Autodesk Fusion 360 part; units mm, degrees
(part 2 of 4)
sketch "sketch 3732" plane through (0, 0, 0) normal (0, 1, 0) x (1, 0, 0)
  arc A0 (-1.8258, -74.9829) -> (1.8258, -74.9829) centre (0, 0) ccw
  arc A1 (9.805, -63.395) -> (9.351, -63.0605) centre (9.4097, -63.4561) ccw
  line L0 (4.6702, -65.7139) -> (4.5475, -63.9874)
  arc A2 (14.9052, -73.5092) -> (18.4653, -72.6966) centre (0, 0) ccw
  spline S0 degree 3 poles (4.376, -68.1369) (4.6576, -66.7896) (4.6745, -65.9819) (4.6702, -65.7139) knots 0 0 0 0 1 1 1 1
  line L1 (9.805, -63.395) -> (10.0696, -65.1055)
  spline S1 degree 3 poles (10.8935, -67.4001) (11.5834, -68.8958) (12.799, -71.009) (14.9052, -73.5092) knots 0 0 0 0 1 1 1 1
  spline S2 degree 3 poles (10.0696, -65.1055) (10.1251, -65.3677) (10.3212, -66.1515) (10.8935, -67.4001) knots 0 0 0 0 1 1 1 1
  arc A3 (4.9157, -63.5602) -> (9.351, -63.0605) centre (0, 0) ccw
  spline S3 degree 3 poles (-4.3775, -68.1342) (-4.0378, -69.746) (-3.3229, -72.0767) (-1.8258, -74.9829) knots 0 0 0 0 1 1 1 1
  spline S4 degree 3 poles (1.8258, -74.9829) (3.3229, -72.0767) (4.0378, -69.746) (4.376, -68.1369) knots 0 0 0 0 1 1 1 1
  arc A4 (4.9157, -63.5602) -> (4.5475, -63.9874) centre (4.9465, -63.959) ccw
  arc A5 (45.3236, -59.7623) -> (48.1785, -57.4856) centre (0, 0) ccw
  spline S5 degree 3 poles (19.4282, -65.4548) (19.403, -64.0786) (19.2396, -63.2874) (19.1758, -63.0271) knots 0 0 0 0 1 1 1 1
  arc A6 (43.4724, -46.6285) -> (46.6285, -43.4724) centre (0, 0) ccw
  spline S6 degree 3 poles (48.4653, -44.6233) (48.6722, -44.7937) (49.3142, -45.2841) (50.5402, -45.9035) knots 0 0 0 0 1 1 1 1
  arc A7 (18.9359, -60.8728) -> (18.672, -61.3711) centre (19.0547, -61.2547) ccw
  line L2 (32.7199, -57.1798) -> (31.8603, -55.6775)
  line L3 (47.192, -43.4509) -> (48.4653, -44.6233)
  spline S7 degree 3 poles (50.5402, -45.9035) (52.0121, -46.6428) (54.28, -47.537) (57.4856, -48.1785) knots 0 0 0 0 1 1 1 1
  arc A8 (57.4856, -48.1785) -> (59.7623, -45.3236) centre (0, 0) ccw
  line L4 (55.6775, -31.8603) -> (57.1798, -32.7199)
  spline S8 degree 3 poles (24.3045, -61.2325) (24.4169, -61.4758) (24.7825, -62.1962) (25.6183, -63.2862) knots 0 0 0 0 1 1 1 1
  arc A9 (30.8888, -68.3494) -> (34.1789, -66.765) centre (0, 0) ccw
  arc A10 (18.9359, -60.8728) -> (23.1489, -59.3986) centre (0, 0) ccw
  line L5 (23.6659, -59.6237) -> (24.3045, -61.2325)
  spline S9 degree 3 poles (25.6183, -63.2862) (26.6237, -64.5909) (28.2791, -66.3806) (30.8888, -68.3494) knots 0 0 0 0 1 1 1 1
  spline S10 degree 3 poles (18.4653, -72.6966) (19.2781, -69.5301) (19.4565, -67.0988) (19.4282, -65.4548) knots 0 0 0 0 1 1 1 1
  spline S11 degree 3 poles (34.1789, -66.765) (34.2667, -63.4971) (33.8996, -61.087) (33.5061, -59.4906) knots 0 0 0 0 1 1 1 1
  arc A11 (36.3401, -52.8627) -> (35.7859, -52.7582) centre (36.0104, -53.0893) ccw
  spline S12 degree 3 poles (39.0585, -55.9988) (40.329, -57.0472) (42.3411, -58.4236) (45.3236, -59.7623) knots 0 0 0 0 1 1 1 1
  arc A12 (47.192, -43.4509) -> (46.6285, -43.4724) centre (46.9211, -43.7451) ccw
  spline S13 degree 3 poles (37.3206, -54.289) (37.4844, -54.5012) (38.0011, -55.1222) (39.0585, -55.9988) knots 0 0 0 0 1 1 1 1
  arc A13 (32.0066, -55.1329) -> (35.7859, -52.7582) centre (0, 0) ccw
  line L6 (44.6233, -48.4653) -> (43.4509, -47.192)
  arc A14 (43.4724, -46.6285) -> (43.4509, -47.192) centre (43.7451, -46.9211) ccw
  spline S14 degree 3 poles (48.1785, -57.4856) (47.537, -54.28) (46.6428, -52.0121) (45.904, -50.5432) knots 0 0 0 0 1 1 1 1
  line L7 (19.1758, -63.0271) -> (18.672, -61.3711)
  arc A15 (23.6659, -59.6237) -> (23.1489, -59.3986) centre (23.2941, -59.7713) ccw
  arc A16 (32.0066, -55.1329) -> (31.8603, -55.6775) centre (32.2074, -55.4789) ccw
  spline S15 degree 3 poles (33.5061, -59.4906) (33.1753, -58.1545) (32.84, -57.4195) (32.7199, -57.1798) knots 0 0 0 0 1 1 1 1
  line L8 (36.3401, -52.8627) -> (37.3206, -54.289)
  spline S16 degree 3 poles (45.904, -50.5432) (45.2841, -49.3142) (44.7937, -48.6722) (44.6233, -48.4653) knots 0 0 0 0 1 1 1 1
  line L9 (54.289, -37.3206) -> (52.8627, -36.3401)
  spline S17 degree 3 poles (59.4875, -33.5063) (61.087, -33.8996) (63.4971, -34.2667) (66.765, -34.1789) knots 0 0 0 0 1 1 1 1
  spline S18 degree 3 poles (68.3494, -30.8888) (66.3806, -28.2791) (64.5909, -26.6237) (63.2879, -25.6209) knots 0 0 0 0 1 1 1 1
  arc A17 (59.3986, -23.1489) -> (60.8728, -18.9359) centre (0, 0) ccw
  line L10 (61.2325, -24.3045) -> (59.6237, -23.6659)
  line L11 (61.3711, -18.672) -> (63.0271, -19.1758)
  spline S19 degree 3 poles (56, -39.0614) (55.1222, -38.0011) (54.5012, -37.4844) (54.289, -37.3206) knots 0 0 0 0 1 1 1 1
  spline S20 degree 3 poles (63.0271, -19.1758) (63.2874, -19.2396) (64.0786, -19.403) (65.4519, -19.4291) knots 0 0 0 0 1 1 1 1
  spline S21 degree 3 poles (65.4519, -19.4291) (67.0988, -19.4565) (69.5301, -19.2781) (72.6966, -18.4653) knots 0 0 0 0 1 1 1 1
  arc A18 (72.6966, -18.4653) -> (73.5092, -14.9052) centre (0, 0) ccw
  arc A19 (63.0605, -9.351) -> (63.5602, -4.9157) centre (0, 0) ccw
  arc A20 (52.7582, -35.7859) -> (55.1329, -32.0066) centre (0, 0) ccw
  arc A21 (63.0605, -9.351) -> (63.395, -9.805) centre (63.4561, -9.4097) ccw
  arc A22 (52.7582, -35.7859) -> (52.8627, -36.3401) centre (53.0893, -36.0104) ccw
  line L12 (65.1055, -10.0696) -> (63.395, -9.805)
  spline S22 degree 3 poles (59.7623, -45.3236) (58.4236, -42.3411) (57.0472, -40.329) (56, -39.0614) knots 0 0 0 0 1 1 1 1
  arc A23 (55.6775, -31.8603) -> (55.1329, -32.0066) centre (55.4789, -32.2074) ccw
  spline S23 degree 3 poles (57.1798, -32.7199) (57.4195, -32.84) (58.1545, -33.1753) (59.4875, -33.5063) knots 0 0 0 0 1 1 1 1
  spline S24 degree 3 poles (63.2879, -25.6209) (62.1962, -24.7825) (61.4758, -24.4169) (61.2325, -24.3045) knots 0 0 0 0 1 1 1 1
  arc A24 (66.765, -34.1789) -> (68.3494, -30.8888) centre (0, 0) ccw
  arc A25 (59.3986, -23.1489) -> (59.6237, -23.6659) centre (59.7713, -23.2941) ccw
  arc A26 (61.3711, -18.672) -> (60.8728, -18.9359) centre (61.2547, -19.0547) ccw
  spline S25 degree 3 poles (-10.0696, 65.1055) (-10.1251, 65.3677) (-10.3212, 66.1515) (-10.8935, 67.4001) knots 0 0 0 0 1 1 1 1
  spline S26 degree 3 poles (19.1758, 63.0271) (19.2396, 63.2874) (19.403, 64.0786) (19.4291, 65.4519) knots 0 0 0 0 1 1 1 1
  arc A27 (9.351, 63.0605) -> (4.9157, 63.5602) centre (0, 0) ccw
  arc A28 (-36.3401, 52.8627) -> (-35.7859, 52.7582) centre (-36.0104, 53.0893) ccw
  line L13 (-32.7199, 57.1798) -> (-31.8603, 55.6775)
  arc A29 (-9.805, 63.395) -> (-9.351, 63.0605) centre (-9.4097, 63.4561) ccw
  arc A30 (-32.0066, 55.1329) -> (-31.8603, 55.6775) centre (-32.2074, 55.4789) ccw
  arc A31 (34.1789, 66.765) -> (30.8888, 68.3494) centre (0, 0) ccw
  spline S27 degree 3 poles (-10.8935, 67.4001) (-11.5834, 68.8958) (-12.799, 71.009) (-14.9052, 73.5092) knots 0 0 0 0 1 1 1 1
  arc A32 (18.672, 61.3711) -> (18.9359, 60.8728) centre (19.0547, 61.2547) ccw
  line L14 (-4.6702, 65.7139) -> (-4.5475, 63.9874)
  arc A33 (-18.9359, 60.8728) -> (-23.1489, 59.3986) centre (0, 0) ccw
  spline S28 degree 3 poles (19.4291, 65.4519) (19.4565, 67.0988) (19.2781, 69.5301) (18.4653, 72.6966) knots 0 0 0 0 1 1 1 1
  spline S29 degree 3 poles (-34.1789, 66.765) (-34.2667, 63.4971) (-33.8996, 61.087) (-33.5061, 59.4906) knots 0 0 0 0 1 1 1 1
  arc A34 (-45.3236, 59.7623) -> (-48.1785, 57.4856) centre (0, 0) ccw
  spline S30 degree 3 poles (-45.904, 50.5432) (-45.2841, 49.3142) (-44.7937, 48.6722) (-44.6233, 48.4653) knots 0 0 0 0 1 1 1 1
  arc A35 (-14.9052, 73.5092) -> (-18.4653, 72.6966) centre (0, 0) ccw
  spline S31 degree 3 poles (10.8956, 67.4023) (10.3212, 66.1515) (10.1251, 65.3677) (10.0696, 65.1055) knots 0 0 0 0 1 1 1 1
  spline S32 degree 3 poles (14.9052, 73.5092) (12.799, 71.009) (11.5834, 68.8958) (10.8956, 67.4023) knots 0 0 0 0 1 1 1 1
  spline S33 degree 3 poles (-37.3206, 54.289) (-37.4844, 54.5012) (-38.0011, 55.1222) (-39.0585, 55.9988) knots 0 0 0 0 1 1 1 1
  spline S34 degree 3 poles (-1.8258, 74.9829) (-3.3229, 72.0767) (-4.0378, 69.746) (-4.376, 68.1369) knots 0 0 0 0 1 1 1 1
  line L15 (-47.192, 43.4509) -> (-48.4653, 44.6233)
  arc A36 (-43.4724, 46.6285) -> (-46.6285, 43.4724) centre (0, 0) ccw
  arc A37 (-47.192, 43.4509) -> (-46.6285, 43.4724) centre (-46.9211, 43.7451) ccw
  spline S35 degree 3 poles (-18.4653, 72.6966) (-19.2781, 69.5301) (-19.4565, 67.0988) (-19.4282, 65.4548) knots 0 0 0 0 1 1 1 1
  spline S36 degree 3 poles (4.3775, 68.1342) (4.0378, 69.746) (3.3229, 72.0767) (1.8258, 74.9829) knots 0 0 0 0 1 1 1 1
  arc A38 (23.1489, 59.3986) -> (23.6659, 59.6237) centre (23.2941, 59.7713) ccw
  line L16 (4.5475, 63.9874) -> (4.6702, 65.7139)
  spline S37 degree 3 poles (-33.5061, 59.4906) (-33.1753, 58.1545) (-32.84, 57.4195) (-32.7199, 57.1798) knots 0 0 0 0 1 1 1 1
  arc A39 (4.5475, 63.9874) -> (4.9157, 63.5602) centre (4.9465, 63.959) ccw
  spline S38 degree 3 poles (-24.3045, 61.2325) (-24.4169, 61.4758) (-24.7825, 62.1962) (-25.6183, 63.2862) knots 0 0 0 0 1 1 1 1
  circle A40 centre (0, 0) radius 4
  arc A41 (-4.9157, 63.5602) -> (-4.5475, 63.9874) centre (-4.9465, 63.959) ccw
  arc A42 (-32.0066, 55.1329) -> (-35.7859, 52.7582) centre (0, 0) ccw
  line L17 (-36.3401, 52.8627) -> (-37.3206, 54.289)
  spline S39 degree 3 poles (-39.0585, 55.9988) (-40.329, 57.0472) (-42.3411, 58.4236) (-45.3236, 59.7623) knots 0 0 0 0 1 1 1 1
  spline S40 degree 3 poles (33.5063, 59.4875) (33.8996, 61.087) (34.2667, 63.4971) (34.1789, 66.765) knots 0 0 0 0 1 1 1 1
  arc A43 (-23.6659, 59.6237) -> (-23.1489, 59.3986) centre (-23.2941, 59.7713) ccw
  arc A44 (-30.8888, 68.3494) -> (-34.1789, 66.765) centre (0, 0) ccw
  arc A45 (-18.9359, 60.8728) -> (-18.672, 61.3711) centre (-19.0547, 61.2547) ccw
  arc A46 (23.1489, 59.3986) -> (18.9359, 60.8728) centre (0, 0) ccw
  arc A47 (-4.9157, 63.5602) -> (-9.351, 63.0605) centre (0, 0) ccw
  spline S41 degree 3 poles (-25.6183, 63.2862) (-26.6237, 64.5909) (-28.2791, 66.3806) (-30.8888, 68.3494) knots 0 0 0 0 1 1 1 1
  line L18 (-19.1758, 63.0271) -> (-18.672, 61.3711)
  line L19 (18.672, 61.3711) -> (19.1758, 63.0271)
  arc A48 (-43.4724, 46.6285) -> (-43.4509, 47.192) centre (-43.7451, 46.9211) ccw
  line L20 (-44.6233, 48.4653) -> (-43.4509, 47.192)
  line L21 (24.3045, 61.2325) -> (23.6659, 59.6237)
  spline S42 degree 3 poles (4.6702, 65.7139) (4.6745, 65.9819) (4.6576, 66.7896) (4.3775, 68.1342) knots 0 0 0 0 1 1 1 1
  spline S43 degree 3 poles (-4.376, 68.1369) (-4.6576, 66.7896) (-4.6745, 65.9819) (-4.6702, 65.7139) knots 0 0 0 0 1 1 1 1
  spline S44 degree 3 poles (-19.4282, 65.4548) (-19.403, 64.0786) (-19.2396, 63.2874) (-19.1758, 63.0271) knots 0 0 0 0 1 1 1 1
  spline S45 degree 3 poles (-48.1785, 57.4856) (-47.537, 54.28) (-46.6428, 52.0121) (-45.904, 50.5432) knots 0 0 0 0 1 1 1 1
  spline S46 degree 3 poles (67.4023, -10.8956) (66.1515, -10.3212) (65.3677, -10.1251) (65.1055, -10.0696) knots 0 0 0 0 1 1 1 1
  arc A49 (18.4653, 72.6966) -> (14.9052, 73.5092) centre (0, 0) ccw
  line L22 (-9.805, 63.395) -> (-10.0696, 65.1055)
  line L23 (10.0696, 65.1055) -> (9.805, 63.395)
  spline S47 degree 3 poles (-4.6702, -65.7139) (-4.6745, -65.9819) (-4.6576, -66.7896) (-4.3775, -68.1342) knots 0 0 0 0 1 1 1 1
  arc A50 (9.351, 63.0605) -> (9.805, 63.395) centre (9.4097, 63.4561) ccw
  spline S48 degree 3 poles (30.8888, 68.3494) (28.2791, 66.3806) (26.6237, 64.5909) (25.6209, 63.2879) knots 0 0 0 0 1 1 1 1
  spline S49 degree 3 poles (32.7199, 57.1798) (32.84, 57.4195) (33.1753, 58.1545) (33.5063, 59.4875) knots 0 0 0 0 1 1 1 1
  line L24 (-23.6659, 59.6237) -> (-24.3045, 61.2325)
  spline S50 degree 3 poles (25.6209, 63.2879) (24.7825, 62.1962) (24.4169, 61.4758) (24.3045, 61.2325) knots 0 0 0 0 1 1 1 1
  spline S51 degree 3 poles (73.5092, -14.9052) (71.009, -12.799) (68.8958, -11.5834) (67.4023, -10.8956) knots 0 0 0 0 1 1 1 1
  arc A51 (1.8258, 74.9829) -> (-1.8258, 74.9829) centre (0, 0) ccw
  spline S52 degree 3 poles (-68.1369, -4.376) (-66.7896, -4.6576) (-65.9819, -4.6745) (-65.7139, -4.6702) knots 0 0 0 0 1 1 1 1
  line L25 (-63.395, -9.805) -> (-65.1055, -10.0696)
  arc A52 (-63.0605, 9.351) -> (-63.5602, 4.9157) centre (0, 0) ccw
  arc A53 (-59.6237, -23.6659) -> (-59.3986, -23.1489) centre (-59.7713, -23.2941) ccw
  arc A54 (-55.1329, -32.0066) -> (-52.7582, -35.7859) centre (0, 0) ccw
  arc A55 (-52.8627, -36.3401) -> (-52.7582, -35.7859) centre (-53.0893, -36.0104) ccw
  line L26 (-52.8627, -36.3401) -> (-54.289, -37.3206)
  spline S53 degree 3 poles (-65.4519, 19.4291) (-67.0988, 19.4565) (-69.5301, 19.2781) (-72.6966, 18.4653) knots 0 0 0 0 1 1 1 1
  spline S54 degree 3 poles (-73.5092, 14.9052) (-71.009, 12.799) (-68.8958, 11.5834) (-67.4023, 10.8956) knots 0 0 0 0 1 1 1 1
  arc A56 (-52.7582, 35.7859) -> (-55.1329, 32.0066) centre (0, 0) ccw
  line L27 (-65.7139, -4.6702) -> (-63.9874, -4.5475)
  arc A57 (-57.4856, 48.1785) -> (-59.7623, 45.3236) centre (0, 0) ccw
  arc A58 (-59.3986, 23.1489) -> (-59.6237, 23.6659) centre (-59.7713, 23.2941) ccw
  spline S55 degree 3 poles (-63.2879, 25.6209) (-62.1962, 24.7825) (-61.4758, 24.4169) (-61.2325, 24.3045) knots 0 0 0 0 1 1 1 1
  line L28 (-61.3711, 18.672) -> (-63.0271, 19.1758)
  spline S56 degree 3 poles (-54.289, -37.3206) (-54.5012, -37.4844) (-55.1222, -38.0011) (-55.9988, -39.0585) knots 0 0 0 0 1 1 1 1
  arc A59 (-59.7623, -45.3236) -> (-57.4856, -48.1785) centre (0, 0) ccw
  spline S57 degree 3 poles (-55.9988, -39.0585) (-57.0472, -40.329) (-58.4236, -42.3411) (-59.7623, -45.3236) knots 0 0 0 0 1 1 1 1
  arc A60 (-63.0605, 9.351) -> (-63.395, 9.805) centre (-63.4561, 9.4097) ccw
  spline S58 degree 3 poles (-65.1055, -10.0696) (-65.3677, -10.1251) (-66.1515, -10.3212) (-67.4001, -10.8935) knots 0 0 0 0 1 1 1 1
  arc A61 (-61.3711, 18.672) -> (-60.8728, 18.9359) centre (-61.2547, 19.0547) ccw
  spline S59 degree 3 poles (-63.0271, 19.1758) (-63.2874, 19.2396) (-64.0786, 19.403) (-65.4519, 19.4291) knots 0 0 0 0 1 1 1 1
  spline S60 degree 3 poles (-59.4875, 33.5063) (-61.087, 33.8996) (-63.4971, 34.2667) (-66.765, 34.1789) knots 0 0 0 0 1 1 1 1
  spline S61 degree 3 poles (-50.5402, 45.9035) (-52.0121, 46.6428) (-54.28, 47.537) (-57.4856, 48.1785) knots 0 0 0 0 1 1 1 1
  line L29 (-61.2325, 24.3045) -> (-59.6237, 23.6659)
  arc A62 (-55.6775, 31.8603) -> (-55.1329, 32.0066) centre (-55.4789, 32.2074) ccw
  spline S62 degree 3 poles (-65.7139, 4.6702) (-65.9819, 4.6745) (-66.7896, 4.6576) (-68.1342, 4.3775) knots 0 0 0 0 1 1 1 1
  arc A63 (-63.395, -9.805) -> (-63.0605, -9.351) centre (-63.4561, -9.4097) ccw
  line L30 (-65.1055, 10.0696) -> (-63.395, 9.805)
  spline S63 degree 3 poles (-67.4023, 10.8956) (-66.1515, 10.3212) (-65.3677, 10.1251) (-65.1055, 10.0696) knots 0 0 0 0 1 1 1 1
  arc A64 (-63.9874, 4.5475) -> (-63.5602, 4.9157) centre (-63.959, 4.9465) ccw
  arc A65 (-63.5602, -4.9157) -> (-63.0605, -9.351) centre (0, 0) ccw
  spline S64 degree 3 poles (-68.1342, 4.3775) (-69.746, 4.0378) (-72.0767, 3.3229) (-74.9829, 1.8258) knots 0 0 0 0 1 1 1 1
  line L31 (-63.9874, 4.5475) -> (-65.7139, 4.6702)
  line L32 (-57.1798, -32.7199) -> (-55.6775, -31.8603)
  spline S65 degree 3 poles (-66.765, -34.1789) (-63.4971, -34.2667) (-61.087, -33.8996) (-59.4906, -33.5061) knots 0 0 0 0 1 1 1 1
  arc A66 (-63.5602, -4.9157) -> (-63.9874, -4.5475) centre (-63.959, -4.9465) ccw
  arc A67 (-66.765, 34.1789) -> (-68.3494, 30.8888) centre (0, 0) ccw
  arc A68 (-60.8728, -18.9359) -> (-61.3711, -18.672) centre (-61.2547, -19.0547) ccw
  spline S66 degree 3 poles (-48.4653, 44.6233) (-48.6722, 44.7937) (-49.3142, 45.2841) (-50.5402, 45.9035) knots 0 0 0 0 1 1 1 1
  arc A69 (-60.8728, -18.9359) -> (-59.3986, -23.1489) centre (0, 0) ccw
  line L33 (-54.289, 37.3206) -> (-52.8627, 36.3401)
  spline S67 degree 3 poles (-72.6966, -18.4653) (-69.5301, -19.2781) (-67.0988, -19.4565) (-65.4548, -19.4282) knots 0 0 0 0 1 1 1 1
  arc A70 (-52.7582, 35.7859) -> (-52.8627, 36.3401) centre (-53.0893, 36.0104) ccw
  arc A71 (-73.5092, -14.9052) -> (-72.6966, -18.4653) centre (0, 0) ccw
  spline S68 degree 3 poles (-57.1798, 32.7199) (-57.4195, 32.84) (-58.1545, 33.1753) (-59.4875, 33.5063) knots 0 0 0 0 1 1 1 1
  line L34 (-59.6237, -23.6659) -> (-61.2325, -24.3045)
  arc A72 (-72.6966, 18.4653) -> (-73.5092, 14.9052) centre (0, 0) ccw
  spline S69 degree 3 poles (-74.9829, -1.8258) (-72.0767, -3.3229) (-69.746, -4.0378) (-68.1369, -4.376) knots 0 0 0 0 1 1 1 1
  line L35 (-55.6775, 31.8603) -> (-57.1798, 32.7199)
  spline S70 degree 3 poles (-67.4001, -10.8935) (-68.8958, -11.5834) (-71.009, -12.799) (-73.5092, -14.9052) knots 0 0 0 0 1 1 1 1
  spline S71 degree 3 poles (-56, 39.0614) (-55.1222, 38.0011) (-54.5012, 37.4844) (-54.289, 37.3206) knots 0 0 0 0 1 1 1 1
  spline S72 degree 3 poles (-65.4548, -19.4282) (-64.0786, -19.403) (-63.2874, -19.2396) (-63.0271, -19.1758) knots 0 0 0 0 1 1 1 1
  arc A73 (-74.9829, 1.8258) -> (-74.9829, -1.8258) centre (0, 0) ccw
  line L36 (-63.0271, -19.1758) -> (-61.3711, -18.672)
  arc A74 (-68.3494, -30.8888) -> (-66.765, -34.1789) centre (0, 0) ccw
  spline S73 degree 3 poles (-59.7623, 45.3236) (-58.4236, 42.3411) (-57.0472, 40.329) (-56, 39.0614) knots 0 0 0 0 1 1 1 1
  spline S74 degree 3 poles (-63.2862, -25.6183) (-64.5909, -26.6237) (-66.3806, -28.2791) (-68.3494, -30.8888) knots 0 0 0 0 1 1 1 1
  spline S75 degree 3 poles (-61.2325, -24.3045) (-61.4758, -24.4169) (-62.1962, -24.7825) (-63.2862, -25.6183) knots 0 0 0 0 1 1 1 1
  spline S76 degree 3 poles (-59.4906, -33.5061) (-58.1545, -33.1753) (-57.4195, -32.84) (-57.1798, -32.7199) knots 0 0 0 0 1 1 1 1
  arc A75 (-55.1329, -32.0066) -> (-55.6775, -31.8603) centre (-55.4789, -32.2074) ccw
  spline S77 degree 3 poles (-68.3494, 30.8888) (-66.3806, 28.2791) (-64.5909, 26.6237) (-63.2879, 25.6209) knots 0 0 0 0 1 1 1 1
  arc A76 (-59.3986, 23.1489) -> (-60.8728, 18.9359) centre (0, 0) ccw
  spline S78 degree 3 poles (-14.9052, -73.5092) (-12.799, -71.009) (-11.5834, -68.8958) (-10.8956, -67.4023) knots 0 0 0 0 1 1 1 1
  spline S79 degree 3 poles (45.3236, 59.7623) (42.3411, 58.4236) (40.329, 57.0472) (39.0614, 56) knots 0 0 0 0 1 1 1 1
  spline S80 degree 3 poles (-33.5063, -59.4875) (-33.8996, -61.087) (-34.2667, -63.4971) (-34.1789, -66.765) knots 0 0 0 0 1 1 1 1
  arc A77 (35.7859, 52.7582) -> (32.0066, 55.1329) centre (0, 0) ccw
  spline S81 degree 3 poles (50.5432, 45.904) (49.3142, 45.2841) (48.6722, 44.7937) (48.4653, 44.6233) knots 0 0 0 0 1 1 1 1
  spline S82 degree 3 poles (65.1055, 10.0696) (65.3677, 10.1251) (66.1515, 10.3212) (67.4001, 10.8935) knots 0 0 0 0 1 1 1 1
  arc A78 (63.5602, 4.9157) -> (63.9874, 4.5475) centre (63.959, 4.9465) ccw
  line L37 (37.3206, 54.289) -> (36.3401, 52.8627)
  arc A79 (-46.6285, -43.4724) -> (-47.192, -43.4509) centre (-46.9211, -43.7451) ccw
  arc A80 (-9.351, -63.0605) -> (-9.805, -63.395) centre (-9.4097, -63.4561) ccw
  line L38 (-10.0696, -65.1055) -> (-9.805, -63.395)
  spline S83 degree 3 poles (68.1342, -4.3775) (69.746, -4.0378) (72.0767, -3.3229) (74.9829, -1.8258) knots 0 0 0 0 1 1 1 1
  spline S84 degree 3 poles (68.1369, 4.376) (66.7896, 4.6576) (65.9819, 4.6745) (65.7139, 4.6702) knots 0 0 0 0 1 1 1 1
  arc A81 (63.5602, 4.9157) -> (63.0605, 9.351) centre (0, 0) ccw
  spline S85 degree 3 poles (74.9829, 1.8258) (72.0767, 3.3229) (69.746, 4.0378) (68.1369, 4.376) knots 0 0 0 0 1 1 1 1
  line L39 (63.9874, -4.5475) -> (65.7139, -4.6702)
  line L40 (-43.4509, -47.192) -> (-44.6233, -48.4653)
  spline S86 degree 3 poles (-45.3236, -59.7623) (-42.3411, -58.4236) (-40.329, -57.0472) (-39.0614, -56) knots 0 0 0 0 1 1 1 1
  arc A82 (-34.1789, -66.765) -> (-30.8888, -68.3494) centre (0, 0) ccw
  spline S87 degree 3 poles (39.0614, 56) (38.0011, 55.1222) (37.4844, 54.5012) (37.3206, 54.289) knots 0 0 0 0 1 1 1 1
  spline S88 degree 3 poles (44.6233, 48.4653) (44.7937, 48.6722) (45.2841, 49.3142) (45.9035, 50.5402) knots 0 0 0 0 1 1 1 1
  spline S89 degree 3 poles (57.4856, 48.1785) (54.28, 47.537) (52.0121, 46.6428) (50.5432, 45.904) knots 0 0 0 0 1 1 1 1
  line L41 (43.4509, 47.192) -> (44.6233, 48.4653)
  line L42 (-24.3045, -61.2325) -> (-23.6659, -59.6237)
  arc A83 (46.6285, 43.4724) -> (43.4724, 46.6285) centre (0, 0) ccw
  spline S90 degree 3 poles (-50.5432, -45.904) (-49.3142, -45.2841) (-48.6722, -44.7937) (-48.4653, -44.6233) knots 0 0 0 0 1 1 1 1
  spline S91 degree 3 poles (-44.6233, -48.4653) (-44.7937, -48.6722) (-45.2841, -49.3142) (-45.9035, -50.5402) knots 0 0 0 0 1 1 1 1
  line L43 (-37.3206, -54.289) -> (-36.3401, -52.8627)
  spline S92 degree 3 poles (-30.8888, -68.3494) (-28.2791, -66.3806) (-26.6237, -64.5909) (-25.6209, -63.2879) knots 0 0 0 0 1 1 1 1
  line L44 (-31.8603, -55.6775) -> (-32.7199, -57.1798)
  line L45 (31.8603, 55.6775) -> (32.7199, 57.1798)
  arc A84 (-4.5475, -63.9874) -> (-4.9157, -63.5602) centre (-4.9465, -63.959) ccw
  arc A85 (-31.8603, -55.6775) -> (-32.0066, -55.1329) centre (-32.2074, -55.4789) ccw
  line L46 (-18.672, -61.3711) -> (-19.1758, -63.0271)
  arc A86 (46.6285, 43.4724) -> (47.192, 43.4509) centre (46.9211, 43.7451) ccw
  arc A87 (-48.1785, -57.4856) -> (-45.3236, -59.7623) centre (0, 0) ccw
  arc A88 (-18.672, -61.3711) -> (-18.9359, -60.8728) centre (-19.0547, -61.2547) ccw
  spline S93 degree 3 poles (45.9035, 50.5402) (46.6428, 52.0121) (47.537, 54.28) (48.1785, 57.4856) knots 0 0 0 0 1 1 1 1
  arc A89 (35.7859, 52.7582) -> (36.3401, 52.8627) centre (36.0104, 53.0893) ccw
  line L47 (-4.5475, -63.9874) -> (-4.6702, -65.7139)
  spline S94 degree 3 poles (-57.4856, -48.1785) (-54.28, -47.537) (-52.0121, -46.6428) (-50.5432, -45.904) knots 0 0 0 0 1 1 1 1
  arc A90 (-23.1489, -59.3986) -> (-18.9359, -60.8728) centre (0, 0) ccw
  arc A91 (63.9874, -4.5475) -> (63.5602, -4.9157) centre (63.959, -4.9465) ccw
  spline S95 degree 3 poles (65.7139, -4.6702) (65.9819, -4.6745) (66.7896, -4.6576) (68.1342, -4.3775) knots 0 0 0 0 1 1 1 1
  spline S96 degree 3 poles (-32.7199, -57.1798) (-32.84, -57.4195) (-33.1753, -58.1545) (-33.5063, -59.4875) knots 0 0 0 0 1 1 1 1
  arc A92 (74.9829, -1.8258) -> (74.9829, 1.8258) centre (0, 0) ccw
  spline S97 degree 3 poles (-25.6209, -63.2879) (-24.7825, -62.1962) (-24.4169, -61.4758) (-24.3045, -61.2325) knots 0 0 0 0 1 1 1 1
  arc A93 (-46.6285, -43.4724) -> (-43.4724, -46.6285) centre (0, 0) ccw
  spline S98 degree 3 poles (-45.9035, -50.5402) (-46.6428, -52.0121) (-47.537, -54.28) (-48.1785, -57.4856) knots 0 0 0 0 1 1 1 1
  arc A94 (-43.4509, -47.192) -> (-43.4724, -46.6285) centre (-43.7451, -46.9211) ccw
  arc A95 (-23.1489, -59.3986) -> (-23.6659, -59.6237) centre (-23.2941, -59.7713) ccw
  spline S99 degree 3 poles (-19.1758, -63.0271) (-19.2396, -63.2874) (-19.403, -64.0786) (-19.4291, -65.4519) knots 0 0 0 0 1 1 1 1
  spline S100 degree 3 poles (-19.4291, -65.4519) (-19.4565, -67.0988) (-19.2781, -69.5301) (-18.4653, -72.6966) knots 0 0 0 0 1 1 1 1
  spline S101 degree 3 poles (-10.8956, -67.4023) (-10.3212, -66.1515) (-10.1251, -65.3677) (-10.0696, -65.1055) knots 0 0 0 0 1 1 1 1
  spline S102 degree 3 poles (-39.0614, -56) (-38.0011, -55.1222) (-37.4844, -54.5012) (-37.3206, -54.289) knots 0 0 0 0 1 1 1 1
  arc A96 (-18.4653, -72.6966) -> (-14.9052, -73.5092) centre (0, 0) ccw
  arc A97 (-9.351, -63.0605) -> (-4.9157, -63.5602) centre (0, 0) ccw
  arc A98 (-35.7859, -52.7582) -> (-36.3401, -52.8627) centre (-36.0104, -53.0893) ccw
  arc A99 (31.8603, 55.6775) -> (32.0066, 55.1329) centre (32.2074, 55.4789) ccw
  line L48 (48.4653, 44.6233) -> (47.192, 43.4509)
  arc A100 (43.4509, 47.192) -> (43.4724, 46.6285) centre (43.7451, 46.9211) ccw
  arc A101 (48.1785, 57.4856) -> (45.3236, 59.7623) centre (0, 0) ccw
  line L49 (-48.4653, -44.6233) -> (-47.192, -43.4509)
  arc A102 (-35.7859, -52.7582) -> (-32.0066, -55.1329) centre (0, 0) ccw
  spline S103 degree 3 poles (63.2862, 25.6183) (64.5909, 26.6237) (66.3806, 28.2791) (68.3494, 30.8888) knots 0 0 0 0 1 1 1 1
  arc A103 (63.395, 9.805) -> (63.0605, 9.351) centre (63.4561, 9.4097) ccw
  arc A104 (52.8627, 36.3401) -> (52.7582, 35.7859) centre (53.0893, 36.0104) ccw
  spline S104 degree 3 poles (66.765, 34.1789) (63.4971, 34.2667) (61.087, 33.8996) (59.4906, 33.5061) knots 0 0 0 0 1 1 1 1
  line L50 (59.6237, 23.6659) -> (61.2325, 24.3045)
  spline S105 degree 3 poles (59.4906, 33.5061) (58.1545, 33.1753) (57.4195, 32.84) (57.1798, 32.7199) knots 0 0 0 0 1 1 1 1
  arc A105 (73.5092, 14.9052) -> (72.6966, 18.4653) centre (0, 0) ccw
  line L51 (63.0271, 19.1758) -> (61.3711, 18.672)
  spline S106 degree 3 poles (54.289, 37.3206) (54.5012, 37.4844) (55.1222, 38.0011) (55.9988, 39.0585) knots 0 0 0 0 1 1 1 1
  line L52 (52.8627, 36.3401) -> (54.289, 37.3206)
  arc A106 (60.8728, 18.9359) -> (59.3986, 23.1489) centre (0, 0) ccw
  line L53 (63.395, 9.805) -> (65.1055, 10.0696)
  spline S107 degree 3 poles (55.9988, 39.0585) (57.0472, 40.329) (58.4236, 42.3411) (59.7623, 45.3236) knots 0 0 0 0 1 1 1 1
  spline S108 degree 3 poles (65.4548, 19.4282) (64.0786, 19.403) (63.2874, 19.2396) (63.0271, 19.1758) knots 0 0 0 0 1 1 1 1
  spline S109 degree 3 poles (61.2325, 24.3045) (61.4758, 24.4169) (62.1962, 24.7825) (63.2862, 25.6183) knots 0 0 0 0 1 1 1 1
  arc A107 (59.6237, 23.6659) -> (59.3986, 23.1489) centre (59.7713, 23.2941) ccw
  arc A108 (55.1329, 32.0066) -> (55.6775, 31.8603) centre (55.4789, 32.2074) ccw
  arc A109 (55.1329, 32.0066) -> (52.7582, 35.7859) centre (0, 0) ccw
  arc A110 (60.8728, 18.9359) -> (61.3711, 18.672) centre (61.2547, 19.0547) ccw
  arc A111 (59.7623, 45.3236) -> (57.4856, 48.1785) centre (0, 0) ccw
  spline S110 degree 3 poles (67.4001, 10.8935) (68.8958, 11.5834) (71.009, 12.799) (73.5092, 14.9052) knots 0 0 0 0 1 1 1 1
  spline S111 degree 3 poles (72.6966, 18.4653) (69.5301, 19.2781) (67.0988, 19.4565) (65.4548, 19.4282) knots 0 0 0 0 1 1 1 1
  line L54 (65.7139, 4.6702) -> (63.9874, 4.5475)
  line L55 (57.1798, 32.7199) -> (55.6775, 31.8603)
  arc A112 (68.3494, 30.8888) -> (66.765, 34.1789) centre (0, 0) ccw
extrude "Extrude1'" add sketch "sketch 3732" along normal blind 8 separate body makes body 2 in component "Spur Gear (28 teeth)"
sketch "Sketch1 (2)" plane through (0, 0, 0) normal (0, 1, 0) x (1, 0, 0) in component "Spur Gear (28 teeth)"
  circle A0 centre (0, 0) radius 70 construction
sketch "sketch 19514" plane through (0, 0, 0) normal (0, 1, 0) x (1, 0, 0)
  spline S0 degree 3 poles (255.5218, 110.66) (257.638, 110.8195) (259.9728, 110.9211) (262.5234, 110.9347) knots 0 0 0 0 1 1 1 1
  arc A0 (258.8882, 96.3563) -> (259.2799, 96.0962) centre (259.2631, 96.4958) ccw
  spline S1 degree 3 poles (264.2658, 87.7533) (263.7058, 87.324) (263.1597, 86.9156) (262.6282, 86.5274) knots 0 0 0 0 1 1 1 1
  arc A1 (253.0782, 110.7207) -> (251.1958, 114.9274) centre (0, 0) ccw
  arc A2 (264.0748, 107.1894) -> (262.5234, 110.9347) centre (0, 0) ccw
  spline S2 degree 3 poles (266.3051, 81.3548) (268.4259, 81.2764) (270.7574, 81.1159) (273.2935, 80.8439) knots 0 0 0 0 1 1 1 1
  arc A3 (268.0489, 66.7641) -> (268.409, 66.4618) centre (268.437, 66.8608) ccw
  arc A4 (278.2986, 61.4407) -> (277.3965, 65.393) centre (0, 0) ccw
  arc A5 (271.3707, 51.6295) -> (270.4716, 56.1496) centre (0, 0) ccw
  spline S3 degree 3 poles (246.8902, 124.5221) (247.5406, 124.6234) (248.2155, 124.7208) (248.9151, 124.8131) knots 0 0 0 0 1 1 1 1
  arc A6 (271.3707, 51.6295) -> (271.7132, 51.3074) centre (271.7636, 51.7042) ccw
  arc A7 (262.6282, 86.5274) -> (262.4841, 86.0798) centre (262.8642, 86.2044) ccw
  spline S4 degree 3 poles (272.4294, 57.6132) (271.8248, 57.2492) (271.2365, 56.9046) (270.6648, 56.5783) knots 0 0 0 0 1 1 1 1
  arc A8 (-107.1894, 264.0748) -> (-110.9347, 262.5234) centre (0, 0) ccw
  spline S5 degree 3 poles (-110.66, 255.5218) (-110.8195, 257.638) (-110.9211, 259.9728) (-110.9347, 262.5234) knots 0 0 0 0 1 1 1 1
  spline S6 degree 3 poles (268.409, 66.4618) (269.0656, 66.4158) (269.7452, 66.3606) (270.4478, 66.295) knots 0 0 0 0 1 1 1 1
  spline S7 degree 3 poles (-107.1894, 264.0748) (-105.3955, 262.2616) (-103.8164, 260.5388) (-102.4328, 258.9296) knots 0 0 0 0 1 1 1 1
  spline S8 degree 3 poles (-102.4328, 258.9296) (-101.9727, 258.3946) (-101.5344, 257.8723) (-101.1169, 257.3634) knots 0 0 0 0 1 1 1 1
  spline S9 degree 3 poles (241.5251, 138.5736) (243.6102, 138.969) (245.919, 139.3314) (248.452, 139.6305) knots 0 0 0 0 1 1 1 1
  spline S10 degree 3 poles (259.2799, 96.0962) (259.9375, 96.124) (260.6191, 96.1452) (261.3246, 96.1587) knots 0 0 0 0 1 1 1 1
  arc A9 (257.3634, 101.1169) -> (257.2447, 100.662) centre (257.6171, 100.8077) ccw
  arc A10 (267.0666, 71.6656) -> (266.8977, 71.2268) centre (267.2842, 71.3299) ccw
  spline S11 degree 3 poles (268.7704, 72.7978) (268.1872, 72.4005) (267.6191, 72.0234) (267.0666, 71.6656) knots 0 0 0 0 1 1 1 1
  spline S12 degree 3 poles (245.8327, 130.7796) (245.3526, 130.2625) (244.8826, 129.7685) (244.4236, 129.2967) knots 0 0 0 0 1 1 1 1
  spline S13 degree 3 poles (261.3246, 96.1587) (263.4464, 96.1992) (265.7832, 96.1698) (268.3306, 96.0404) knots 0 0 0 0 1 1 1 1
  spline S14 degree 3 poles (269.6695, 92.214) (267.7586, 90.5246) (265.9499, 89.0445) (264.2658, 87.7533) knots 0 0 0 0 1 1 1 1
  spline S15 degree 3 poles (271.7132, 51.3074) (272.3662, 51.2247) (273.0417, 51.1315) (273.7395, 51.0266) knots 0 0 0 0 1 1 1 1
  spline S16 degree 3 poles (278.2986, 61.4407) (276.2105, 59.9759) (274.2475, 58.7077) (272.4294, 57.6132) knots 0 0 0 0 1 1 1 1
  arc A11 (-101.1169, 257.3634) -> (-100.662, 257.2447) centre (-100.8077, 257.6171) ccw
  arc A12 (-96.3563, 258.8882) -> (-100.662, 257.2447) centre (0, 0) ccw
  arc A13 (250.4129, 136.0824) -> (248.452, 139.6305) centre (0, 0) ccw
  arc A14 (246.4719, 124.7367) -> (246.8902, 124.5221) centre (246.8288, 124.9173) ccw
  arc A15 (246.4719, 124.7367) -> (244.3566, 128.8313) centre (0, 0) ccw
  spline S17 degree 3 poles (253.4839, 110.4829) (254.1389, 110.5476) (254.8182, 110.607) (255.5218, 110.66) knots 0 0 0 0 1 1 1 1
  spline S18 degree 3 poles (250.4129, 136.0824) (248.812, 134.0968) (247.2768, 132.3347) (245.8327, 130.7796) knots 0 0 0 0 1 1 1 1
  arc A16 (253.0782, 110.7207) -> (253.4839, 110.4829) centre (253.4447, 110.881) ccw
  arc A17 (251.2888, 115.3883) -> (251.1958, 114.9274) centre (251.5595, 115.0938) ccw
  spline S19 degree 3 poles (264.0748, 107.1894) (262.2616, 105.3955) (260.5388, 103.8164) (258.9296, 102.4328) knots 0 0 0 0 1 1 1 1
  arc A18 (269.6695, 92.214) -> (268.3306, 96.0404) centre (0, 0) ccw
  spline S20 degree 3 poles (258.9296, 102.4328) (258.3946, 101.9727) (257.8723, 101.5344) (257.3634, 101.1169) knots 0 0 0 0 1 1 1 1
  arc A19 (263.8837, 81.6887) -> (264.2602, 81.407) centre (264.2658, 81.807) ccw
  spline S21 degree 3 poles (257.6492, 121.8275) (255.9395, 119.9348) (254.3079, 118.2616) (252.7789, 116.7899) knots 0 0 0 0 1 1 1 1
  arc A20 (274.4157, 76.9484) -> (273.2935, 80.8439) centre (0, 0) ccw
  spline S22 degree 3 poles (264.2602, 81.407) (264.9183, 81.398) (265.6, 81.381) (266.3051, 81.3548) knots 0 0 0 0 1 1 1 1
  spline S23 degree 3 poles (274.4157, 76.9484) (272.4131, 75.3688) (270.5243, 73.9925) (268.7704, 72.7978) knots 0 0 0 0 1 1 1 1
  arc A21 (270.6648, 56.5783) -> (270.4716, 56.1496) centre (270.8632, 56.2309) ccw
  spline S24 degree 3 poles (270.4478, 66.295) (272.5608, 66.0977) (274.8797, 65.8068) (277.3965, 65.393) knots 0 0 0 0 1 1 1 1
  spline S25 degree 3 poles (252.7789, 116.7899) (252.2705, 116.3006) (251.7735, 115.8336) (251.2888, 115.3883) knots 0 0 0 0 1 1 1 1
  arc A22 (258.8882, 96.3563) -> (257.2447, 100.662) centre (0, 0) ccw
  arc A23 (257.6492, 121.8275) -> (255.8902, 125.48) centre (0, 0) ccw
  arc A24 (244.4236, 129.2967) -> (244.3566, 128.8313) centre (244.7104, 129.0178) ccw
  spline S26 degree 3 poles (248.9151, 124.8131) (251.019, 125.091) (253.3445, 125.3234) (255.8902, 125.48) knots 0 0 0 0 1 1 1 1
  arc A25 (263.8837, 81.6887) -> (262.4841, 86.0798) centre (0, 0) ccw
  arc A26 (268.0489, 66.7641) -> (266.8977, 71.2268) centre (0, 0) ccw
  arc A27 (-76.9484, 274.4157) -> (-80.8439, 273.2935) centre (0, 0) ccw
  spline S27 degree 3 poles (-96.1587, 261.3246) (-96.1992, 263.4464) (-96.1698, 265.7832) (-96.0404, 268.3306) knots 0 0 0 0 1 1 1 1
  spline S28 degree 3 poles (-66.4618, 268.409) (-66.4158, 269.0656) (-66.3606, 269.7452) (-66.295, 270.4478) knots 0 0 0 0 1 1 1 1
  spline S29 degree 3 poles (-45.7398, 281.3058) (-44.3943, 279.1389) (-43.2382, 277.1078) (-42.2473, 275.2312) knots 0 0 0 0 1 1 1 1
  arc A28 (-29.8949, 283.4279) -> (-33.9233, 282.974) centre (0, 0) ccw
  arc A29 (-71.6656, 267.0666) -> (-71.2268, 266.8977) centre (-71.3299, 267.2842) ccw
  spline S30 degree 3 poles (-66.295, 270.4478) (-66.0977, 272.5608) (-65.8068, 274.8797) (-65.393, 277.3965) knots 0 0 0 0 1 1 1 1
  spline S31 degree 3 poles (-20.5626, 275.7494) (-20.4073, 276.389) (-20.239, 277.0498) (-20.0566, 277.7315) knots 0 0 0 0 1 1 1 1
  arc A30 (-41.313, 273.4114) -> (-40.8958, 273.1944) centre (-40.9551, 273.59) ccw
  spline S32 degree 3 poles (-35.9916, 274.1626) (-35.8724, 274.81) (-35.7415, 275.4792) (-35.5976, 276.1699) knots 0 0 0 0 1 1 1 1
  arc A31 (-20.921, 275.445) -> (-25.5134, 275.0576) centre (0, 0) ccw
  spline S33 degree 3 poles (-20.0566, 277.7315) (-19.5082, 279.7816) (-18.833, 282.0189) (-18.0035, 284.4309) knots 0 0 0 0 1 1 1 1
  arc A32 (-10.4408, 276.3178) -> (-10.0506, 276.0555) centre (-10.0652, 276.4552) ccw
  arc A33 (-5.4437, 276.1847) -> (-10.0506, 276.0555) centre (0, 0) ccw
  arc A34 (-5.4437, 276.1847) -> (-5.0688, 276.4685) centre (-5.4516, 276.5847) ccw
  arc A35 (-13.9559, 284.6582) -> (-18.0035, 284.4309) centre (0, 0) ccw
  spline S34 degree 3 poles (-13.9559, 284.6582) (-12.8615, 282.3543) (-11.94, 280.2066) (-11.1655, 278.2308) knots 0 0 0 0 1 1 1 1
  spline S35 degree 3 poles (-4.4526, 278.4191) (-3.79, 280.4352) (-2.9904, 282.6312) (-2.027, 284.9929) knots 0 0 0 0 1 1 1 1
  arc A36 (-20.921, 275.445) -> (-20.5626, 275.7494) centre (-20.9513, 275.8439) ccw
  spline S36 degree 3 poles (-57.6132, 272.4294) (-57.2492, 271.8248) (-56.9046, 271.2365) (-56.5783, 270.6648) knots 0 0 0 0 1 1 1 1
  arc A37 (2.027, 284.9929) -> (-2.027, 284.9929) centre (0, 0) ccw
  spline S37 degree 3 poles (-5.0688, 276.4685) (-4.8779, 277.0984) (-4.6729, 277.7488) (-4.4526, 278.4191) knots 0 0 0 0 1 1 1 1
  spline S38 degree 3 poles (-51.0266, 273.7395) (-50.7111, 275.8381) (-50.2907, 278.137) (-49.7364, 280.6267) knots 0 0 0 0 1 1 1 1
  arc A38 (10.0506, 276.0555) -> (10.4408, 276.3178) centre (10.0652, 276.4552) ccw
  arc A39 (-45.7398, 281.3058) -> (-49.7364, 280.6267) centre (0, 0) ccw
  arc A40 (-86.5274, 262.6282) -> (-86.0798, 262.4841) centre (-86.2044, 262.8642) ccw
  arc A41 (-61.4407, 278.2986) -> (-65.393, 277.3965) centre (0, 0) ccw
  arc A42 (-36.3324, 273.8386) -> (-40.8958, 273.1944) centre (0, 0) ccw
  arc A43 (-25.9177, 275.2977) -> (-25.5134, 275.0576) centre (-25.5503, 275.4559) ccw
  arc A44 (-81.6887, 263.8837) -> (-81.407, 264.2602) centre (-81.807, 264.2658) ccw
  arc A45 (-81.6887, 263.8837) -> (-86.0798, 262.4841) centre (0, 0) ccw
  spline S39 degree 3 poles (-81.3548, 266.3051) (-81.2764, 268.4259) (-81.1159, 270.7574) (-80.8439, 273.2935) knots 0 0 0 0 1 1 1 1
  arc A46 (-96.3563, 258.8882) -> (-96.0962, 259.2799) centre (-96.4958, 259.2631) ccw
  spline S40 degree 3 poles (-81.407, 264.2602) (-81.398, 264.9183) (-81.381, 265.6) (-81.3548, 266.3051) knots 0 0 0 0 1 1 1 1
  arc A47 (-51.6295, 271.3707) -> (-51.3074, 271.7132) centre (-51.7042, 271.7636) ccw
  arc A48 (-92.214, 269.6695) -> (-96.0404, 268.3306) centre (0, 0) ccw
  spline S41 degree 3 poles (-72.7978, 268.7704) (-72.4005, 268.1872) (-72.0234, 267.6191) (-71.6656, 267.0666) knots 0 0 0 0 1 1 1 1
  spline S42 degree 3 poles (-61.4407, 278.2986) (-59.9759, 276.2105) (-58.7077, 274.2475) (-57.6132, 272.4294) knots 0 0 0 0 1 1 1 1
  arc A49 (-36.3324, 273.8386) -> (-35.9916, 274.1626) centre (-36.385, 274.2352) ccw
  spline S43 degree 3 poles (-42.2473, 275.2312) (-41.9178, 274.6072) (-41.6067, 274.0004) (-41.313, 273.4114) knots 0 0 0 0 1 1 1 1
  spline S44 degree 3 poles (-11.1655, 278.2308) (-10.908, 277.5738) (-10.6668, 276.936) (-10.4408, 276.3178) knots 0 0 0 0 1 1 1 1
  arc A50 (-66.7641, 268.0489) -> (-71.2268, 266.8977) centre (0, 0) ccw
  spline S45 degree 3 poles (-51.3074, 271.7132) (-51.2247, 272.3662) (-51.1315, 273.0417) (-51.0266, 273.7395) knots 0 0 0 0 1 1 1 1
  spline S46 degree 3 poles (-87.7533, 264.2658) (-87.324, 263.7058) (-86.9156, 263.1597) (-86.5274, 262.6282) knots 0 0 0 0 1 1 1 1
  spline S47 degree 3 poles (-92.214, 269.6695) (-90.5246, 267.7586) (-89.0445, 265.9499) (-87.7533, 264.2658) knots 0 0 0 0 1 1 1 1
  spline S48 degree 3 poles (-96.0962, 259.2799) (-96.124, 259.9375) (-96.1452, 260.6191) (-96.1587, 261.3246) knots 0 0 0 0 1 1 1 1
  spline S49 degree 3 poles (-29.8949, 283.4279) (-28.673, 281.1889) (-27.6326, 279.0963) (-26.7485, 277.167) knots 0 0 0 0 1 1 1 1
  spline S50 degree 3 poles (-26.7485, 277.167) (-26.4545, 276.5255) (-26.1779, 275.9023) (-25.9177, 275.2977) knots 0 0 0 0 1 1 1 1
  spline S51 degree 3 poles (-76.9484, 274.4157) (-75.3688, 272.4131) (-73.9925, 270.5243) (-72.7978, 268.7704) knots 0 0 0 0 1 1 1 1
  arc A51 (-66.7641, 268.0489) -> (-66.4618, 268.409) centre (-66.8608, 268.437) ccw
  arc A52 (-56.5783, 270.6648) -> (-56.1496, 270.4716) centre (-56.2309, 270.8632) ccw
  arc A53 (-51.6295, 271.3707) -> (-56.1496, 270.4716) centre (0, 0) ccw
  spline S52 degree 3 poles (-35.5976, 276.1699) (-35.165, 278.2476) (-34.6163, 280.5193) (-33.9233, 282.974) knots 0 0 0 0 1 1 1 1
  arc A54 (35.9916, 274.1626) -> (36.3324, 273.8386) centre (36.385, 274.2352) ccw
  arc A55 (71.2268, 266.8977) -> (66.7641, 268.0489) centre (0, 0) ccw
  spline S53 degree 3 poles (71.6656, 267.0666) (72.0234, 267.6191) (72.4005, 268.1872) (72.7978, 268.7704) knots 0 0 0 0 1 1 1 1
  spline S54 degree 3 poles (102.4328, 258.9296) (103.8164, 260.5388) (105.3955, 262.2616) (107.1894, 264.0748) knots 0 0 0 0 1 1 1 1
  spline S55 degree 3 poles (26.7485, 277.167) (27.6326, 279.0963) (28.673, 281.1889) (29.8949, 283.4279) knots 0 0 0 0 1 1 1 1
  spline S56 degree 3 poles (42.2473, 275.2312) (43.2382, 277.1078) (44.3943, 279.1389) (45.7398, 281.3058) knots 0 0 0 0 1 1 1 1
  spline S57 degree 3 poles (51.0266, 273.7395) (51.1315, 273.0417) (51.2247, 272.3662) (51.3074, 271.7132) knots 0 0 0 0 1 1 1 1
  arc A56 (5.0688, 276.4685) -> (5.4437, 276.1847) centre (5.4516, 276.5847) ccw
  arc A57 (80.8439, 273.2935) -> (76.9484, 274.4157) centre (0, 0) ccw
  spline S58 degree 3 poles (35.5976, 276.1699) (35.7415, 275.4792) (35.8724, 274.81) (35.9916, 274.1626) knots 0 0 0 0 1 1 1 1
  spline S59 degree 3 poles (4.4526, 278.4191) (4.6729, 277.7488) (4.8779, 277.0984) (5.0688, 276.4685) knots 0 0 0 0 1 1 1 1
  spline S60 degree 3 poles (72.7978, 268.7704) (73.9925, 270.5243) (75.3688, 272.4131) (76.9484, 274.4157) knots 0 0 0 0 1 1 1 1
  spline S61 degree 3 poles (2.027, 284.9929) (2.9904, 282.6312) (3.79, 280.4352) (4.4526, 278.4191) knots 0 0 0 0 1 1 1 1
  arc A58 (56.1496, 270.4716) -> (56.5783, 270.6648) centre (56.2309, 270.8632) ccw
  arc A59 (86.0798, 262.4841) -> (81.6887, 263.8837) centre (0, 0) ccw
  spline S62 degree 3 poles (81.3548, 266.3051) (81.381, 265.6) (81.398, 264.9183) (81.407, 264.2602) knots 0 0 0 0 1 1 1 1
  spline S63 degree 3 poles (101.1169, 257.3634) (101.5344, 257.8723) (101.9727, 258.3946) (102.4328, 258.9296) knots 0 0 0 0 1 1 1 1
  arc A60 (100.662, 257.2447) -> (101.1169, 257.3634) centre (100.8077, 257.6171) ccw
  spline S64 degree 3 poles (96.1587, 261.3246) (96.1452, 260.6191) (96.124, 259.9375) (96.0962, 259.2799) knots 0 0 0 0 1 1 1 1
  arc A61 (51.3074, 271.7132) -> (51.6295, 271.3707) centre (51.7042, 271.7636) ccw
  arc A62 (40.8958, 273.1944) -> (36.3324, 273.8386) centre (0, 0) ccw
  spline S65 degree 3 poles (33.9233, 282.974) (34.6163, 280.5193) (35.165, 278.2476) (35.5976, 276.1699) knots 0 0 0 0 1 1 1 1
  arc A63 (86.0798, 262.4841) -> (86.5274, 262.6282) centre (86.2044, 262.8642) ccw
  spline S66 degree 3 poles (80.8439, 273.2935) (81.1159, 270.7574) (81.2764, 268.4259) (81.3548, 266.3051) knots 0 0 0 0 1 1 1 1
  spline S67 degree 3 poles (41.313, 273.4114) (41.6067, 274.0004) (41.9178, 274.6072) (42.2473, 275.2312) knots 0 0 0 0 1 1 1 1
  arc A64 (40.8958, 273.1944) -> (41.313, 273.4114) centre (40.9551, 273.59) ccw
  arc A65 (71.2268, 266.8977) -> (71.6656, 267.0666) centre (71.3299, 267.2842) ccw
  arc A66 (96.0404, 268.3306) -> (92.214, 269.6695) centre (0, 0) ccw
  spline S68 degree 3 poles (87.7533, 264.2658) (89.0445, 265.9499) (90.5246, 267.7586) (92.214, 269.6695) knots 0 0 0 0 1 1 1 1
  spline S69 degree 3 poles (96.0404, 268.3306) (96.1698, 265.7832) (96.1992, 263.4464) (96.1587, 261.3246) knots 0 0 0 0 1 1 1 1
  arc A67 (96.0962, 259.2799) -> (96.3563, 258.8882) centre (96.4958, 259.2631) ccw
  spline S70 degree 3 poles (11.1655, 278.2308) (11.94, 280.2066) (12.8615, 282.3543) (13.9559, 284.6582) knots 0 0 0 0 1 1 1 1
  arc A68 (25.5134, 275.0576) -> (20.921, 275.445) centre (0, 0) ccw
  spline S71 degree 3 poles (65.393, 277.3965) (65.8068, 274.8797) (66.0977, 272.5608) (66.295, 270.4478) knots 0 0 0 0 1 1 1 1
  spline S72 degree 3 poles (86.5274, 262.6282) (86.9156, 263.1597) (87.324, 263.7058) (87.7533, 264.2658) knots 0 0 0 0 1 1 1 1
  spline S73 degree 3 poles (25.9177, 275.2977) (26.1779, 275.9023) (26.4545, 276.5255) (26.7485, 277.167) knots 0 0 0 0 1 1 1 1
  arc A69 (49.7364, 280.6267) -> (45.7398, 281.3058) centre (0, 0) ccw
  arc A70 (100.662, 257.2447) -> (96.3563, 258.8882) centre (0, 0) ccw
  spline S74 degree 3 poles (18.0035, 284.4309) (18.833, 282.0189) (19.5082, 279.7816) (20.0566, 277.7315) knots 0 0 0 0 1 1 1 1
  arc A71 (20.5626, 275.7494) -> (20.921, 275.445) centre (20.9513, 275.8439) ccw
  spline S75 degree 3 poles (66.295, 270.4478) (66.3606, 269.7452) (66.4158, 269.0656) (66.4618, 268.409) knots 0 0 0 0 1 1 1 1
  arc A72 (18.0035, 284.4309) -> (13.9559, 284.6582) centre (0, 0) ccw
  arc A73 (65.393, 277.3965) -> (61.4407, 278.2986) centre (0, 0) ccw
  arc A74 (81.407, 264.2602) -> (81.6887, 263.8837) centre (81.807, 264.2658) ccw
  arc A75 (110.9347, 262.5234) -> (107.1894, 264.0748) centre (0, 0) ccw
  spline S76 degree 3 poles (110.9347, 262.5234) (110.9211, 259.9728) (110.8195, 257.638) (110.66, 255.5218) knots 0 0 0 0 1 1 1 1
  spline S77 degree 3 poles (10.4408, 276.3178) (10.6668, 276.936) (10.908, 277.5738) (11.1655, 278.2308) knots 0 0 0 0 1 1 1 1
  arc A76 (10.0506, 276.0555) -> (5.4437, 276.1847) centre (0, 0) ccw
  arc A77 (25.5134, 275.0576) -> (25.9177, 275.2977) centre (25.5503, 275.4559) ccw
  arc A78 (66.4618, 268.409) -> (66.7641, 268.0489) centre (66.8608, 268.437) ccw
  arc A79 (33.9233, 282.974) -> (29.8949, 283.4279) centre (0, 0) ccw
  spline S78 degree 3 poles (56.5783, 270.6648) (56.9046, 271.2365) (57.2492, 271.8248) (57.6132, 272.4294) knots 0 0 0 0 1 1 1 1
  spline S79 degree 3 poles (20.0566, 277.7315) (20.239, 277.0498) (20.4073, 276.389) (20.5626, 275.7494) knots 0 0 0 0 1 1 1 1
  spline S80 degree 3 poles (57.6132, 272.4294) (58.7077, 274.2475) (59.9759, 276.2105) (61.4407, 278.2986) knots 0 0 0 0 1 1 1 1
  arc A80 (56.1496, 270.4716) -> (51.6295, 271.3707) centre (0, 0) ccw
  spline S81 degree 3 poles (49.7364, 280.6267) (50.2907, 278.137) (50.7111, 275.8381) (51.0266, 273.7395) knots 0 0 0 0 1 1 1 1
  arc A81 (-124.7367, 246.4719) -> (-128.8313, 244.3566) centre (0, 0) ccw
  spline S82 degree 3 poles (-116.7899, 252.7789) (-116.3006, 252.2705) (-115.8336, 251.7735) (-115.3883, 251.2888) knots 0 0 0 0 1 1 1 1
  arc A82 (-276.0555, 10.0506) -> (-276.3178, 10.4408) centre (-276.4552, 10.0652) ccw
  arc A83 (-276.0555, 10.0506) -> (-276.1847, 5.4437) centre (0, 0) ccw
  arc A84 (-276.4685, 5.0688) -> (-276.1847, 5.4437) centre (-276.5847, 5.4516) ccw
  spline S83 degree 3 poles (-284.4309, 18.0035) (-282.0189, 18.833) (-279.7816, 19.5082) (-277.7315, 20.0566) knots 0 0 0 0 1 1 1 1
  spline S84 degree 3 poles (-276.3178, 10.4408) (-276.936, 10.6668) (-277.5738, 10.908) (-278.2308, 11.1655) knots 0 0 0 0 1 1 1 1
  spline S85 degree 3 poles (-277.7315, 20.0566) (-277.0498, 20.239) (-276.389, 20.4073) (-275.7494, 20.5626) knots 0 0 0 0 1 1 1 1
  arc A85 (124.5221, 246.8902) -> (124.7367, 246.4719) centre (124.9173, 246.8288) ccw
  spline S86 degree 3 poles (130.7796, 245.8327) (132.3347, 247.2768) (134.0968, 248.812) (136.0824, 250.4129) knots 0 0 0 0 1 1 1 1
  spline S87 degree 3 poles (-278.2308, 11.1655) (-280.2066, 11.94) (-282.3543, 12.8615) (-284.6582, 13.9559) knots 0 0 0 0 1 1 1 1
  arc A86 (114.9274, 251.1958) -> (110.7207, 253.0782) centre (0, 0) ccw
  arc A87 (-275.0576, 25.5134) -> (-275.445, 20.921) centre (0, 0) ccw
  arc A88 (-282.974, 33.9233) -> (-283.4279, 29.8949) centre (0, 0) ccw
  spline S88 degree 3 poles (-144.3578, 238.1131) (-143.8146, 237.6627) (-143.295, 237.2212) (-142.7982, 236.7894) knots 0 0 0 0 1 1 1 1
  spline S89 degree 3 poles (-284.9929, 2.027) (-282.6312, 2.9904) (-280.4352, 3.79) (-278.4191, 4.4526) knots 0 0 0 0 1 1 1 1
  arc A89 (128.8313, 244.3566) -> (124.7367, 246.4719) centre (0, 0) ccw
  arc A90 (-275.0576, 25.5134) -> (-275.2977, 25.9177) centre (-275.4559, 25.5503) ccw
  spline S90 degree 3 poles (-277.167, 26.7485) (-279.0963, 27.6326) (-281.1889, 28.673) (-283.4279, 29.8949) knots 0 0 0 0 1 1 1 1
  spline S91 degree 3 poles (-282.974, 33.9233) (-280.5193, 34.6163) (-278.2476, 35.165) (-276.1699, 35.5976) knots 0 0 0 0 1 1 1 1
  spline S92 degree 3 poles (116.7899, 252.7789) (118.2616, 254.3079) (119.9348, 255.9395) (121.8275, 257.6492) knots 0 0 0 0 1 1 1 1
  arc A91 (-142.7982, 236.7894) -> (-142.3298, 236.7485) centre (-142.5359, 237.0914) ccw
  spline S93 degree 3 poles (124.8131, 248.9151) (124.7208, 248.2155) (124.6234, 247.5406) (124.5221, 246.8902) knots 0 0 0 0 1 1 1 1
  spline S94 degree 3 poles (-124.8131, 248.9151) (-125.091, 251.019) (-125.3234, 253.3445) (-125.48, 255.8902) knots 0 0 0 0 1 1 1 1
  spline S95 degree 3 poles (-110.4829, 253.4839) (-110.5476, 254.1389) (-110.607, 254.8182) (-110.66, 255.5218) knots 0 0 0 0 1 1 1 1
  spline S96 degree 3 poles (125.48, 255.8902) (125.3234, 253.3445) (125.091, 251.019) (124.8131, 248.9151) knots 0 0 0 0 1 1 1 1
  arc A92 (-136.0824, 250.4129) -> (-139.6305, 248.452) centre (0, 0) ccw
  spline S97 degree 3 poles (115.3883, 251.2888) (115.8336, 251.7735) (116.3006, 252.2705) (116.7899, 252.7789) knots 0 0 0 0 1 1 1 1
  arc A93 (-284.9929, 2.027) -> (-284.9929, -2.027) centre (0, 0) ccw
  spline S98 degree 3 poles (-275.2977, 25.9177) (-275.9023, 26.1779) (-276.5255, 26.4545) (-277.167, 26.7485) knots 0 0 0 0 1 1 1 1
  spline S99 degree 3 poles (-124.5221, 246.8902) (-124.6234, 247.5406) (-124.7208, 248.2155) (-124.8131, 248.9151) knots 0 0 0 0 1 1 1 1
  spline S100 degree 3 poles (-121.8275, 257.6492) (-119.9348, 255.9395) (-118.2616, 254.3079) (-116.7899, 252.7789) knots 0 0 0 0 1 1 1 1
  arc A94 (-110.7207, 253.0782) -> (-110.4829, 253.4839) centre (-110.881, 253.4447) ccw
  arc A95 (-284.4309, 18.0035) -> (-284.6582, 13.9559) centre (0, 0) ccw
  arc A96 (128.8313, 244.3566) -> (129.2967, 244.4236) centre (129.0178, 244.7104) ccw
  arc A97 (-275.7494, 20.5626) -> (-275.445, 20.921) centre (-275.8439, 20.9513) ccw
  spline S101 degree 3 poles (129.2967, 244.4236) (129.7685, 244.8826) (130.2625, 245.3526) (130.7796, 245.8327) knots 0 0 0 0 1 1 1 1
  spline S102 degree 3 poles (-130.7796, 245.8327) (-130.2625, 245.3526) (-129.7685, 244.8826) (-129.2967, 244.4236) knots 0 0 0 0 1 1 1 1
  arc A98 (-124.7367, 246.4719) -> (-124.5221, 246.8902) centre (-124.9173, 246.8288) ccw
  arc A99 (125.48, 255.8902) -> (121.8275, 257.6492) centre (0, 0) ccw
  spline S103 degree 3 poles (-276.4685, -5.0688) (-277.0984, -4.8779) (-277.7488, -4.6729) (-278.4191, -4.4526) knots 0 0 0 0 1 1 1 1
  spline S104 degree 3 poles (-278.4191, 4.4526) (-277.7488, 4.6729) (-277.0984, 4.8779) (-276.4685, 5.0688) knots 0 0 0 0 1 1 1 1
  spline S105 degree 3 poles (-138.5736, 241.5251) (-138.969, 243.6102) (-139.3314, 245.919) (-139.6305, 248.452) knots 0 0 0 0 1 1 1 1
  arc A100 (114.9274, 251.1958) -> (115.3883, 251.2888) centre (115.0938, 251.5595) ccw
  arc A101 (-138.3603, 239.0901) -> (-138.1694, 239.5198) centre (-138.5606, 239.4363) ccw
  arc A102 (-138.3603, 239.0901) -> (-142.3298, 236.7485) centre (0, 0) ccw
  spline S106 degree 3 poles (110.66, 255.5218) (110.607, 254.8182) (110.5476, 254.1389) (110.4829, 253.4839) knots 0 0 0 0 1 1 1 1
  spline S107 degree 3 poles (-138.1694, 239.5198) (-138.307, 240.1635) (-138.4421, 240.8319) (-138.5736, 241.5251) knots 0 0 0 0 1 1 1 1
  arc A103 (-121.8275, 257.6492) -> (-125.48, 255.8902) centre (0, 0) ccw
  arc A104 (-110.7207, 253.0782) -> (-114.9274, 251.1958) centre (0, 0) ccw
  spline S108 degree 3 poles (-278.4191, -4.4526) (-280.4352, -3.79) (-282.6312, -2.9904) (-284.9929, -2.027) knots 0 0 0 0 1 1 1 1
  arc A105 (-129.2967, 244.4236) -> (-128.8313, 244.3566) centre (-129.0178, 244.7104) ccw
  arc A106 (-115.3883, 251.2888) -> (-114.9274, 251.1958) centre (-115.0938, 251.5595) ccw
  arc A107 (110.4829, 253.4839) -> (110.7207, 253.0782) centre (110.881, 253.4447) ccw
  arc A108 (139.6305, 248.452) -> (136.0824, 250.4129) centre (0, 0) ccw
  spline S109 degree 3 poles (-149.9091, 242.3888) (-147.8368, 240.9017) (-145.9914, 239.4677) (-144.3578, 238.1131) knots 0 0 0 0 1 1 1 1
  spline S110 degree 3 poles (-136.0824, 250.4129) (-134.0968, 248.812) (-132.3347, 247.2768) (-130.7796, 245.8327) knots 0 0 0 0 1 1 1 1
  arc A109 (-266.8977, 71.2268) -> (-268.0489, 66.7641) centre (0, 0) ccw
  spline S111 degree 3 poles (-262.5234, 110.9347) (-259.9728, 110.9211) (-257.638, 110.8195) (-255.5218, 110.66) knots 0 0 0 0 1 1 1 1
  spline S112 degree 3 poles (-277.3965, 65.393) (-274.8797, 65.8068) (-272.5608, 66.0977) (-270.4478, 66.295) knots 0 0 0 0 1 1 1 1